Rim (Autodesk Fusion 360 design; units mm, degrees)
part number: 2026-09-26-21-07-27-495
Autodesk Fusion 360 part; units mm, degrees
sketch "Sketch1" plane through (0, 0, 0) normal (0, 0, 1) x (1, 0, 0)
  line L0 (-86.9849, 25) -> (-86.9849, 125)
  line L1 (-86.9849, 125) -> (-80.4008, 125)
  line L2 (-80.4008, 125) -> (-80.4008, 175)
  line L3 (-80.4008, 175) -> (-40.4008, 175)
  line L4 (-40.4008, 175) -> (-26.2586, 189.1421)
  line L5 (-26.2586, 189.1421) -> (33.7414, 189.1421)
  line L6 (33.7414, 189.1421) -> (71.4286, 219.1421)
  line L7 (71.4286, 219.1421) -> (73.1213, 234.0463)
  line L8 (-85.2557, 180) -> (-42.4718, 180)
  line L9 (-42.4718, 180) -> (-28.3297, 194.1421)
  line L10 (-28.3297, 194.1421) -> (31.9943, 194.1421)
  line L11 (31.9943, 194.1421) -> (66.6943, 221.7642)
  line L12 (66.6943, 221.7642) -> (68.1532, 234.6105)
  line L13 (68.1532, 234.6105) -> (73.1213, 234.0463)
  line L14 (-93.5691, 125) -> (-93.5691, 175)
  line L15 (-242.1231, 234.6105) -> (-247.0911, 234.0463)
  line L16 (-205.9641, 194.1421) -> (-240.6641, 221.7642)
  line L17 (-240.6641, 221.7642) -> (-242.1231, 234.6105)
  line L18 (-145.6402, 194.1421) -> (-205.9641, 194.1421)
  line L19 (-86.9849, 125) -> (-93.5691, 125)
  line L20 (-147.7112, 189.1421) -> (-207.7112, 189.1421)
  line L21 (-93.5691, 175) -> (-133.5691, 175)
  line L22 (-245.3985, 219.1421) -> (-247.0911, 234.0463)
  line L23 (-88.7142, 180) -> (-131.498, 180)
  line L24 (-86.9849, 25) -> (-86.9849, 125)
  line L25 (-131.498, 180) -> (-145.6402, 194.1421)
  line L26 (-133.5691, 175) -> (-147.7112, 189.1421)
  line L27 (-207.7112, 189.1421) -> (-245.3985, 219.1421)
  line L28 (-85.2557, 180) -> (-88.7142, 180)
  line L29 (-86.9849, 25) -> (-270, 25)
  point P0 (-173.9699, 0)
  dimension "d1" = 100
  dimension "d2" = 40
  dimension "d3" = 20
  dimension "d4" = 135
  dimension "d5" = 60
  dimension "d6" = 30
  dimension "d7" = 15
  dimension "d8" = 135
  dimension "d10" = -5
  dimension "d11" = 50
  constraint vertical L0
  constraint perpendicular L0 L1
  constraint perpendicular L1 L2
  constraint perpendicular L2 L3
  constraint perpendicular L2 L5
  constraint perpendicular L7 L13
  constraint symmetric origin L0 P0
  constraint symmetric L24.start L0 L29.start
  constraint symmetric L1.start L0 L19.start
  constraint symmetric L0 L1.end L14.start
  constraint symmetric L0 L2.end L14.end
  constraint symmetric L0 L3.end L21.end
  constraint symmetric L0 L4.end L20.start
  constraint symmetric L0 L5.end L20.end
  constraint symmetric L0 L6.end L22.start
  constraint symmetric L0 L7.end L15.end
  constraint symmetric L0 L8.start L23.start
  constraint symmetric L0 L8.end L23.end
  constraint symmetric L0 L9.end L18.start
  constraint symmetric L0 L10.end L16.start
  constraint symmetric L0 L11.end L16.end
  constraint symmetric L0 L12.end L15.start
  constraint perpendicular L24 L29
  measures "d1" distance of L0.start L0.end
  measures "d2" distance of L2.end L3.end
  measures "d3" distance of L3.end L4.end
  measures "d4" angle of L4 L5
  measures "d5" distance of L4.end L5.end
  measures "d6" vertical distance of L5.end L6.end
  measures "d7" distance of L6.end L7.end
  measures "d8" angle of L6 L7
  measures "d11" distance of L1.end L2.end
revolve "Revolve1" add sketch "Sketch1" angle 360 about axis through (-86.9849, 25, 0) along (-1, 0, 0)
sketch "Sketch2" plane through (-93.5691, 0, 0) normal (-1, 0, 0) x (0, -1, 0)
  circle A0 centre (-25, 0) radius 100
  circle A1 centre (-25, 0) radius 150
  line L0 (-25, 0) -> (-25, -125)
  circle A2 centre (-25, -125) radius 8
  circle A3 centre (37.5, -108.2532) radius 8
  circle A4 centre (83.2532, -62.5) radius 8
  circle A5 centre (100, 0) radius 8
  circle A6 centre (83.2532, 62.5) radius 8
  circle A7 centre (37.5, 108.2532) radius 8
  circle A8 centre (-25, 125) radius 8
  circle A9 centre (-87.5, 108.2532) radius 8
  circle A10 centre (-133.2532, 62.5) radius 8
  circle A11 centre (-150, 0) radius 8
  circle A12 centre (-133.2532, -62.5) radius 8
  circle A13 centre (-87.5, -108.2532) radius 8
  dimension "d13" = 16
  dimension "d15" = 360
  constraint coincident A0.centre A1.centre
  constraint vertical L0
  constraint coincident L0.end A2.centre
  measures "d13" diameter of A2
extrude "Extrude1" cut sketch "Sketch2" against normal blind 200 contours A2 | A3 | A4 | A5 | A6 | A7 | A8 | A9 | A10 | A11 | A12 | A13
